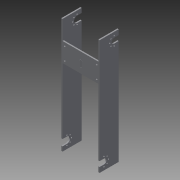
# Autodesk Inventor part: Arm_Third_Flame
Saved by Autodesk Inventor 2013 (Build 170138000, 138)
## iProperties
Created: 2014-04-16
Part Number: Arm_Third_Flame
Material: 一般
Document SubType Name: Modeling
Designer: andou
Density: 1 g/cm^3
Author: andou
Autodesk Inventor part; units mm, degrees
note: some values were not read from the file. Chosen so that the rebuilt part matches the saved one: direction of "エンボス1".
ref_plane "YZ Plane" through (0, 0, 0) normal (1, 0, 0) x (0, 1, 0)
ref_plane "XZ Plane" through (0, 0, 0) normal (0, 1, 0) x (-1, 0, 0)
ref_plane "XY Plane" through (0, 0, 0) normal (0, 0, 1) x (1, 0, 0)
sketch "スケッチ1" plane through (0, 0, 0) normal (0, 0, 1) x (1, 0, 0)
  line L0 (-30, 15) -> (30, 15)
  line L1 (30, 15) -> (30, -15)
  line L2 (30, -15) -> (-30, -15)
  line L3 (-30, -15) -> (-30, 15)
  line L4 (-28, 13) -> (28, 13)
  line L5 (28, 13) -> (28, -13)
  line L6 (28, -13) -> (-28, -13)
  line L7 (-28, -13) -> (-28, 13)
  point P0 (0, 0)
  dimension "d0" = 30
  dimension "d2" = 60
  dimension "d3" = 56
  dimension "d4" = 26
  dimension "d5" = 28
  dimension "d6" = 30
  dimension "d7" = 15
  dimension "d8" = 13
  constraints: 16 end point, 4 parallel, 2 horizontal, 2 perpendicular
  measures "d0" distance of L2.end L0.start
  measures "d2" distance of L0.start L0.end
  measures "d3" distance of L4.start L4.end
  measures "d4" distance of L6.end L4.start
  measures "d5" distance from line of point (0, 0) L7
  measures "d6" distance from line of point (0, 0) L1
  measures "d7" distance from line of point (0, 0) L2
  measures "d8" distance from line of L4 point (0, 0)
extrude "押し出し1" add sketch "スケッチ1" against normal blind 180
sketch "スケッチ8" plane through (-30, 15, 0) normal (0, 1, 0) x (1, 0, 0)
  line L0 (0, 0) -> (60, 0) projected
  line L1 (0, 180) -> (60, 180) projected
  line L2 (0, 0) -> (0, 180) projected
  line L3 (2, 180) -> (58, 180)
  line L4 (58, 180) -> (58, 60)
  line L5 (58, 60) -> (2, 60)
  line L6 (2, 60) -> (2, 180)
  line L7 (2, 0) -> (58, 0)
  line L8 (58, 0) -> (58, 30)
  line L9 (58, 30) -> (2, 30)
  line L10 (2, 30) -> (2, 0)
  point P0 (30, 0)
  dimension "d62" = 56
  dimension "d64" = 2
  dimension "d65" = 2
  dimension "d66" = 56
  dimension "d67" = 30
  dimension "d68" = 120
  constraints: 16 end point, 4 parallel, 2 horizontal, 2 perpendicular, 2 point on line
  measures "d62" distance of L4.end L5.end
  measures "d64" distance between parallel lines of L2 L6
  measures "d65" distance between parallel lines of L2 L10
  measures "d66" distance of L8.end L9.end
  measures "d67" distance of L7.end L8.end
  measures "d68" distance of L3.end L4.end
extrude "押し出し6" cut sketch "スケッチ8" against normal blind 30
sketch "スケッチ9" plane through (30, 15, 0) normal (0, 1, 0) x (1, 0, 0)
  line L0 (-58, 60) -> (-2, 60)
  line L1 (-2, 60) -> (-2, 30)
  line L2 (-2, 30) -> (-58, 30)
  line L3 (-58, 30) -> (-58, 60)
  point P0 (-30, 0)
  constraints: 8 end point, 2 parallel, 1 horizontal, 1 perpendicular
extrude "押し出し7" cut sketch "スケッチ9" against normal blind 2
sketch "スケッチ10" plane through (-30, -15, 0) normal (-1, 0, 0) x (0, 0, 1)
  line L0 (0, 0) -> (0, 30) projected
  line L1 (0, 30) -> (-180, 30) projected
  line L2 (-180, 0) -> (-180, 30) projected
  line L3 (0, 0) -> (-180, 0) projected
  line L4 (-16, 30) -> (-8, 30)
  line L5 (-8, 30) -> (-8, 23)
  line L6 (-16, 23) -> (-16, 30)
  line L7 (-172, 0) -> (-164, 0)
  line L8 (-164, 0) -> (-164, 7)
  line L9 (-172, 7) -> (-172, 0)
  arc A0 (-164, 7) -> (-172, 7) centre (-168, 7) ccw
  arc A1 (-16, 23) -> (-8, 23) centre (-12, 23) ccw
  point P0 (0, 15)
  dimension "d76" = 8
  dimension "d78" = 12
  dimension "d79" = 12
  dimension "d80" = 8
  dimension "d81" = 4
  dimension "d109" = 7
  constraints: 12 end point, 4 point on circle, 3 parallel, 2 centre point, 2 horizontal, 2 perpendicular, 2 point on line, 1 equal radius
  measures "d76" distance between parallel lines of L8 L9
  measures "d78" distance from line of L2 A0.centre
  measures "d79" distance from line of L0 A1.centre
  measures "d80" distance between parallel lines of L5 L6
  measures "d81" radius of A1
  measures "d109" distance from line of A0.centre L3
extrude "押し出し8" cut sketch "スケッチ10" against normal blind 60 contours L3 L9 A0 L8 | L5 A1 L6 L1
sketch "スケッチ11" plane through (-30, -15, 0) normal (-1, 0, 0) x (0, 0, 1)
  line L0 (-16, 23) -> (-16, 30) projected
  line L1 (-16, 30) -> (-180, 30) projected
  line L2 (-172, 0) -> (-180, 0) projected
  line L3 (-172, 0) -> (-172, 7) projected
  arc A0 (-164, 7) -> (-172, 7) centre (-168, 7) ccw projected
  line L4 (-164, 7) -> (-164, 0) projected
  line L5 (0, 0) -> (-164, 0) projected
  line L6 (0, 30) -> (-8, 30) projected
  line L7 (-8, 30) -> (-8, 23) projected
  arc A1 (-16, 23) -> (-8, 23) centre (-12, 23) ccw projected
  arc A2 (-163, 7) -> (-173, 7) centre (-168, 7) ccw
  arc A3 (-17, 23) -> (-7, 23) centre (-12, 23) ccw
  line L8 (-173, 7) -> (-173, 0)
  line L9 (-163, 7) -> (-163, 0)
  line L10 (-17, 23) -> (-17, 30)
  line L11 (-7, 23) -> (-7, 30)
  point P0 (0, 15)
  dimension "d84" = 10
  constraints: 8 end point, 4 point on circle, 4 point on line, 4 tangent, 2 centre point, 2 coincident, 2 parallel, 2 perpendicular, 1 equal radius
  measures "d84" diameter of A2
extrude "押し出し9" cut sketch "スケッチ11" against normal blind 2
sketch "スケッチ12" plane through (-30, -15, 0) normal (-1, 0, 0) x (0, 0, 1)
  line L0 (-173, 0) -> (-180, 0) projected
  arc A0 (-163, 7) -> (-173, 7) centre (-168, 7) ccw projected
  line L1 (0, 30) -> (-7, 30) projected
  arc A1 (-17, 23) -> (-7, 23) centre (-12, 23) ccw projected
  circle A2 centre (-175, 7) radius 1
  circle A3 centre (-5, 23) radius 1
  point P0 (0, 15)
  dimension "d88" = 2
  dimension "d90" = 7
  dimension "d91" = 7
  dimension "d92" = 7
  dimension "d93" = 7
  constraints: 2 centre point, 1 equal radius
  measures "d88" diameter of A2
  measures "d90" distance of A1.centre A3.centre
  measures "d91" distance from line of L1 A3.centre
  measures "d92" distance from line of A2.centre L0
  measures "d93" distance of A0.centre A2.centre
hole "穴3" at (-30, -8, -175) at (-30, 8, -5) direction (1, 0, 0) diameter 2 end through all
pattern_circular "円形状パターン3" count 5 over 180 about axis through (-30, -8, -168) along (1, 0, 0) of "穴3"
pattern_circular "円形状パターン4" count 5 over 180 about axis through (-30, 8, -12) along (1, 0, 0) of "穴3"
sketch "スケッチ13" plane through (-28, -15, -60) normal (0, -1, 0) x (1, 0, 0)
  line L0 (21.928, 20.1792) -> (33.4931, 20.1792) construction
  line L1 (33.4931, 20.1792) -> (33.4931, 9.9574) construction
  line L2 (33.4931, 9.9574) -> (21.928, 9.9574) construction
  line L3 (21.928, 9.9574) -> (21.928, 20.1792) construction
  line L4 (29.3915, 18.4045) -> (29.3915, 8.2019)
  line L5 (29.3915, 8.2019) -> (28.3218, 8.2019)
  line L6 (28.3218, 8.2019) -> (28.3218, 18.4045)
  line L7 (28.3218, 18.4045) -> (26.7092, 17.116)
  line L8 (26.7092, 17.116) -> (26.4904, 17.3348)
  line L9 (26.4904, 17.3348) -> (28.808, 20.1792)
  line L10 (28.808, 20.1792) -> (28.9134, 20.1792)
  line L11 (28.9134, 20.1792) -> (31.2229, 17.3348)
  line L12 (31.2229, 17.3348) -> (31.0041, 17.116)
  line L13 (31.0041, 17.116) -> (29.3915, 18.4045)
  point P0 (28, 60)
  constraints: 2 other
emboss "エンボス1" sketch "スケッチ13" operation cut depth 1 direction (0, 1, 0)
sketch "スケッチ16" plane through (-28, -15, -60) normal (0, -1, 0) x (1, 0, 0)
  line L0 (56, 30) -> (0, 30) projected
  line L1 (-2, 60) -> (-2, -103) projected
  circle A0 centre (3, 25) radius 1.5
  circle A1 centre (3, 5) radius 1.5
  circle A2 centre (53, 5) radius 1.5
  circle A3 centre (53, 25) radius 1.5
  point P0 (28, 60)
  dimension "d128" = 3
  dimension "d131" = 50
  dimension "d132" = 50
  dimension "d133" = 20
  dimension "d134" = 20
  dimension "d135" = 5
  dimension "d136" = 5
  dimension "d137" = 5
  dimension "d138" = 5
  constraints: 4 centre point, 3 equal radius
  measures "d128" diameter of A0
  measures "d131" distance of A3.centre A0.centre
  measures "d132" distance of A2.centre A1.centre
  measures "d133" distance of A0.centre A1.centre
  measures "d134" distance of A3.centre A2.centre
  measures "d135" distance from line of L0 A0.centre
  measures "d136" distance from line of L1 A0.centre
  measures "d137" distance from line of L1 A1.centre
  measures "d138" distance from line of L0 A3.centre
hole "穴4" at (25, -15, -35) at (25, -15, -55) at (-25, -15, -35) at (-25, -15, -55) direction (0, 1, 0) diameter 3 end through all
